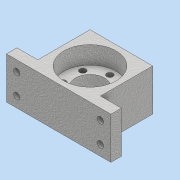
# Autodesk Inventor part: Obudowa nakrętki trapezowej fi 16
Saved by Autodesk Inventor 2018 (Build 220112000, 112)
## iProperties
Created: 2019-01-25
Part Number: Obudowa nakrętki trapezowej fi 16
Material: Ogólny
Document SubType Name: Modeling
Designer: Dawid
Density: 1 g/cm^3
Appearance: Aluminium odlewane
Author: Dawid
Autodesk Inventor part; units mm, degrees
ref_plane "YZ Plane" through (0, 0, 0) normal (1, 0, 0) x (0, 1, 0)
ref_plane "XZ Plane" through (0, 0, 0) normal (0, 1, 0) x (-1, 0, 0)
ref_plane "XY Plane" through (0, 0, 0) normal (0, 0, 1) x (1, 0, 0)
sketch "Szkic1" plane through (0, 0, 0) normal (0, 0, 1) x (1, 0, 0)
  line L0 (-30, -30) -> (30, -30)
  line L1 (30, -30) -> (30, 30)
  line L2 (30, 30) -> (-30, 30)
  line L3 (-30, 30) -> (-30, -30)
  line L4 (-30, -30) -> (30, 30) construction
  line L5 (30, -30) -> (-30, 30) construction
  point P0 (0, 0)
  dimension "d0" = 60
  dimension "d1" = 60
  constraints: 12 end point, 2 midpoint, 2 parallel, 1 horizontal, 1 perpendicular
  measures "d0" distance of L2.end L1.end
  measures "d1" distance of L1.end L0.end
extrude "Wyciągnięcie proste1" add sketch "Szkic1" along normal blind 35
sketch "Szkic2" plane through (0, 0, 35) normal (0, 0, 1) x (1, 0, 0)
  circle A0 centre (0, 0) radius 25
  dimension "d4" = 50
  constraints: 1 centre point, 1 coincident
  measures "d4" diameter of A0
extrude "Wyciągnięcie proste2" cut sketch "Szkic2" against normal blind 12
sketch "Szkic3" plane through (0, 0, 23) normal (0, 0, 1) x (1, 0, 0)
  circle A0 centre (0, 0) radius 14
  dimension "d7" = 28
  constraints: 1 centre point, 1 coincident
  measures "d7" diameter of A0
extrude "Wyciągnięcie proste3" cut sketch "Szkic3" against normal up to next
sketch "Szkic4" plane through (0, 0, 23) normal (0, 0, 1) x (1, 0, 0)
  circle A0 centre (0, 0) radius 19
  circle A1 centre (0, 19) radius 3
  circle A2 centre (-16.4545, 9.5) radius 3
  circle A3 centre (-16.4545, -9.5) radius 3
  circle A4 centre (0, -19) radius 3
  circle A5 centre (16.4545, -9.5) radius 3
  circle A6 centre (16.4545, 9.5) radius 3
  dimension "d10" = 38
  dimension "d11" = 6
  dimension "d14" = 360
  constraints: 6 centre point, 1 coincident, 1 vertical alignment, 15 other
  measures "d11" diameter of A1
extrude "Wyciągnięcie proste4" cut sketch "Szkic4" against normal blind 10 contours A6 A0 | A0 A6 | A5 A0 | A0 A5 | A1 A0 | A0 A1 | A4 A0 | A0 A4 | A2 A0 | A0 A2 | A3 A0 | A0 A3
thread "Gwint1" size "M6x1" class "6H" standard "ANSI Metric M Profile" full length
thread "Gwint2" size "M6x1" class "6H" standard "ANSI Metric M Profile" full length
thread "Gwint3" size "M6x1" class "6H" standard "ANSI Metric M Profile" full length
thread "Gwint4" size "M6x1" class "6H" standard "ANSI Metric M Profile" full length
thread "Gwint5" size "M6x1" class "6H" standard "ANSI Metric M Profile" full length
thread "Gwint6" size "M6x1" class "6H" standard "ANSI Metric M Profile" full length
sketch "Szkic6" plane through (0, 0, 35) normal (0, 0, 1) x (1, 0, 0)
  circle A0 centre (0, 0) radius 25 projected
  line L0 (-30, -30) -> (30, -30) projected
  line L1 (30, -30) -> (30, 30) projected
  line L2 (30, 30) -> (-30, 30) projected
  line L3 (-30, 30) -> (-30, -30) projected
extrude "Wyciągnięcie proste5" add sketch "Szkic6" along normal blind 5
sketch "Szkic8" plane through (30, -30, 0) normal (1, 0, 0) x (0, 0, -1)
  line L0 (0, 0) -> (0, 10)
  line L1 (-40, 0) -> (-40, 10)
  line L2 (0, 0) -> (-40, 0)
  line L3 (-40, 0) -> (-40, 10)
  line L4 (-40, 10) -> (-40, 0)
  line L5 (-40, 10) -> (0, 10)
  point P0 (0, 30)
  dimension "d35" = 10
  constraints: 12 end point
  measures "d35" distance of L1.end L1.start
extrude "Wyciągnięcie proste6" add sketch "Szkic8" along normal blind 20
sketch "Szkic9" plane through (-30, -30, 0) normal (-1, 0, 0) x (0, 0, 1)
  line L0 (0, 10) -> (0, 0)
  line L1 (0, 0) -> (40, 0)
  line L2 (40, 10) -> (40, 0)
  line L3 (0, 0) -> (0, 10)
  line L4 (0, 10) -> (0, 0)
  line L5 (40, 10) -> (0, 10)
  line L6 (0, 10) -> (40, 10)
  line L7 (40, 10) -> (40, 0)
  point P0 (0, 30)
  constraints: 16 end point
extrude "Wyciągnięcie proste7" add sketch "Szkic9" along normal blind 20
sketch "Szkic10" plane through (-30, -20, 40) normal (0, 1, 0) x (1, 0, 0)
  line L0 (0, 40) -> (0, 0) projected
  line L1 (0, 40) -> (-20, 40) projected
  line L2 (-20, 0) -> (-20, 40) projected
  line L3 (0, 0) -> (-20, 0) projected
  line L4 (60, 0) -> (60, 40) projected
  line L5 (60, 0) -> (80, 0) projected
  line L6 (80, 40) -> (80, 0) projected
  line L7 (60, 40) -> (80, 40) projected
  line L8 (-20, 40) -> (80, 40) projected
  line L9 (-20, 40) -> (-10, 40)
  line L10 (80, 40) -> (70, 40)
  line L11 (70, 40) -> (70, 30)
  line L12 (80, 0) -> (70, 0)
  line L13 (80, 0) -> (-20, 0) projected
  line L14 (70, 0) -> (70, 10)
  line L15 (-20, 0) -> (-10, 0)
  line L16 (-10, 0) -> (-10, 10)
  line L17 (-10, 40) -> (-10, 30)
  circle A0 centre (-10, 30) radius 3
  circle A1 centre (-10, 10) radius 3
  circle A2 centre (70, 30) radius 3
  circle A3 centre (70, 10) radius 3
  point P0 (30, 40)
  dimension "d41" = 10
  dimension "d42" = 10
  dimension "d43" = 10
  dimension "d44" = 10
  dimension "d45" = 10
  dimension "d46" = 10
  dimension "d47" = 10
  dimension "d48" = 10
  dimension "d49" = 6
  dimension "d50" = 6
  dimension "d51" = 6
  dimension "d52" = 6
  constraints: 16 end point, 4 centre point, 4 coincident, 4 perpendicular, 4 point on line
  measures "d41" distance of L1.end L9.end
  measures "d42" distance of L6.start L10.end
  measures "d43" distance of L10.end L11.end
  measures "d44" distance of L5.end L12.end
  measures "d45" distance of L12.end L14.end
  measures "d46" distance of L2.start L15.end
  measures "d47" distance of L15.end L16.end
  measures "d48" distance of L9.end L17.end
  measures "d49" diameter of A0
  measures "d50" diameter of A1
  measures "d51" diameter of A2
  measures "d52" diameter of A3
extrude "Wyciągnięcie proste8" cut sketch "Szkic10" against normal up to next contours A0 | A1 | A2 | A3
sketch "Szkic11" plane through (-30, -20, 40) normal (0, 1, 0) x (1, 0, 0)
  circle A0 centre (-10, 30) radius 3 projected
  circle A1 centre (-10, 10) radius 3 projected
  circle A2 centre (70, 10) radius 3 projected
  circle A3 centre (70, 30) radius 3 projected
  circle A4 centre (-10, 30) radius 5
  circle A5 centre (-10, 10) radius 5
  circle A6 centre (70, 30) radius 5
  circle A7 centre (70, 10) radius 5
  point P0 (30, 40)
  dimension "d55" = 10
  dimension "d56" = 10
  dimension "d57" = 10
  dimension "d58" = 10
  constraints: 4 centre point, 4 coincident
  measures "d55" diameter of A4
  measures "d56" diameter of A5
  measures "d57" diameter of A6
  measures "d58" diameter of A7
extrude "Wyciągnięcie proste9" cut sketch "Szkic11" against normal blind 5
